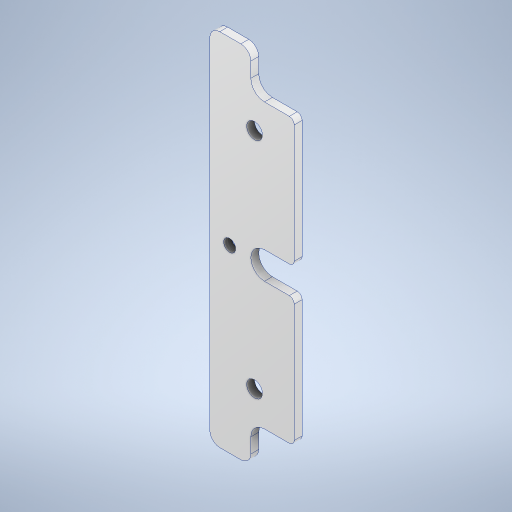
# Autodesk Inventor part: Gantry Belt Retainer
Saved by Autodesk Inventor 2024 (Build 280153000, 153)
## iProperties
Created: 2024-12-26
Part Number: Gantry Belt Retainer
Material: Aluminum 6061
Document SubType Name: Modeling
Designer: Ishaan
Density: 2.7 g/cm^3
Appearance: Aluminum - Flat
Author: Ishaan
Autodesk Inventor part; units mm, degrees
ref_plane "YZ Plane" through (0, 0, 0) normal (1, 0, 0) x (0, 1, 0)
ref_plane "XZ Plane" through (0, 0, 0) normal (0, 1, 0) x (-1, 0, 0)
ref_plane "XY Plane" through (0, 0, 0) normal (0, 0, 1) x (1, 0, 0)
sketch "Sketch1" plane through (0, 0, 0) normal (0, 0, 1) x (1, 0, 0)
  line L0 (8.5, -36.236) -> (-8.5, -36.236)
  line L1 (-8.5, -36.236) -> (-8.5, 36.236)
  line L2 (-8.5, 36.236) -> (8.5, 36.236)
  line L3 (8.5, 36.236) -> (8.5, -36.236)
  line L4 (8.5, -36.236) -> (-8.5, 36.236) construction
  line L5 (-8.5, -36.236) -> (8.5, 36.236) construction
  line L6 (8.5, 0) -> (2.5, 0) construction
  line L7 (8.5, 2.75) -> (2.5, 2.75)
  line L8 (2.5, -2.75) -> (8.5, -2.75)
  arc A0 (8.5, -2.75) -> (8.5, 2.75) centre (8.5, 0) ccw
  arc A1 (2.5, 2.75) -> (2.5, -2.75) centre (2.5, 0) ccw
  line L9 (8.5, 36.236) -> (-0.25, 36.236)
  line L10 (-0.25, 36.236) -> (-0.25, 31.236)
  line L11 (2.5, 28.486) -> (8.5, 28.486)
  line L12 (8.5, 28.486) -> (8.5, 36.236)
  line L13 (8.5, -36.236) -> (-0.25, -36.236)
  line L14 (-0.25, -36.236) -> (-0.25, -31.236)
  line L15 (2.5, -28.486) -> (8.5, -28.486)
  line L16 (8.5, -28.486) -> (8.5, -36.236)
  arc A2 (2.5, -28.486) -> (-0.25, -31.236) centre (2.5, -31.236) ccw
  arc A3 (-0.25, 31.236) -> (2.5, 28.486) centre (2.5, 31.236) ccw
  line L17 (0.5, 22.5) -> (0.5, -22.5) construction
  point P0 (0, 0)
  point P1 (5.5, 0)
  point P2 (0.5, 0)
  point P3 (-8.5, 0)
  point P4 (8.5, -28.486)
  point P5 (8.5, 28.486)
  point P6 (-4.5, 0)
  dimension "d0" = 17
  dimension "d1" = 72.472
  dimension "d3" = 5.5
  dimension "d4" = 11
  dimension "d6" = 5
  dimension "d7" = 5
  dimension "d8" = 45
  dimension "d9" = 9
  dimension "d22" = 4
  constraints: 38 end point, 8 point on circle, 8 tangent, 7 parallel, 6 midpoint, 4 centre point, 4 perpendicular, 3 horizontal, 2 coincident, 2 equal radius, 2 horizontal alignment, 2 vertical alignment, 1 vertical
  measures "d0" distance of L1.end L2.end
  measures "d1" distance of L0.end L1.end
  measures "d3" diameter of A1
  measures "d4" distance from line of L1 L6.end
  measures "d6" distance from line of A2.centre L0
  measures "d7" distance from line of L2 A3.centre
  measures "d8" distance of L17.start L17.end
  measures "d9" distance between parallel lines of L17 L1
  measures "d22" distance of point (-8.5, 0) point (-4.5, 0)
extrude "Extrusion1" add sketch "Sketch1" along normal blind 1.5875 contours L0 L1 L2 L10 A3 L11 L3 L7 A1 L8 L15 A2 L14
fillet "Fillet1" radius 2 2 edges at (-8.5, -36.236, 0.7937) (-8.5, 36.236, 0.7937)
fillet "Fillet2" radius 2 2 edges at (-0.25, -36.236, 0.7937) (-0.25, 36.236, 0.7937)
fillet "Fillet3" radius 1 4 edges at (8.5, -28.486, 0.7937) (8.5, -2.75, 0.7937) (8.5, 2.75, 0.7937) (8.5, 28.486, 0.7937)
hole "Hole1" at (0.5, 22.5, 0) at (0.5, -22.5, 0) direction (0, 0, 1) diameter 3.2 end through all
hole "Hole2" at (-4.5, 0, 0) direction (0, 0, 1) diameter 2.459 end through all thread size "M3x0.5" class "6H" standard "ANSI Metric M Profile"
equation "\"d7\" = d6"
body "Solid1"
